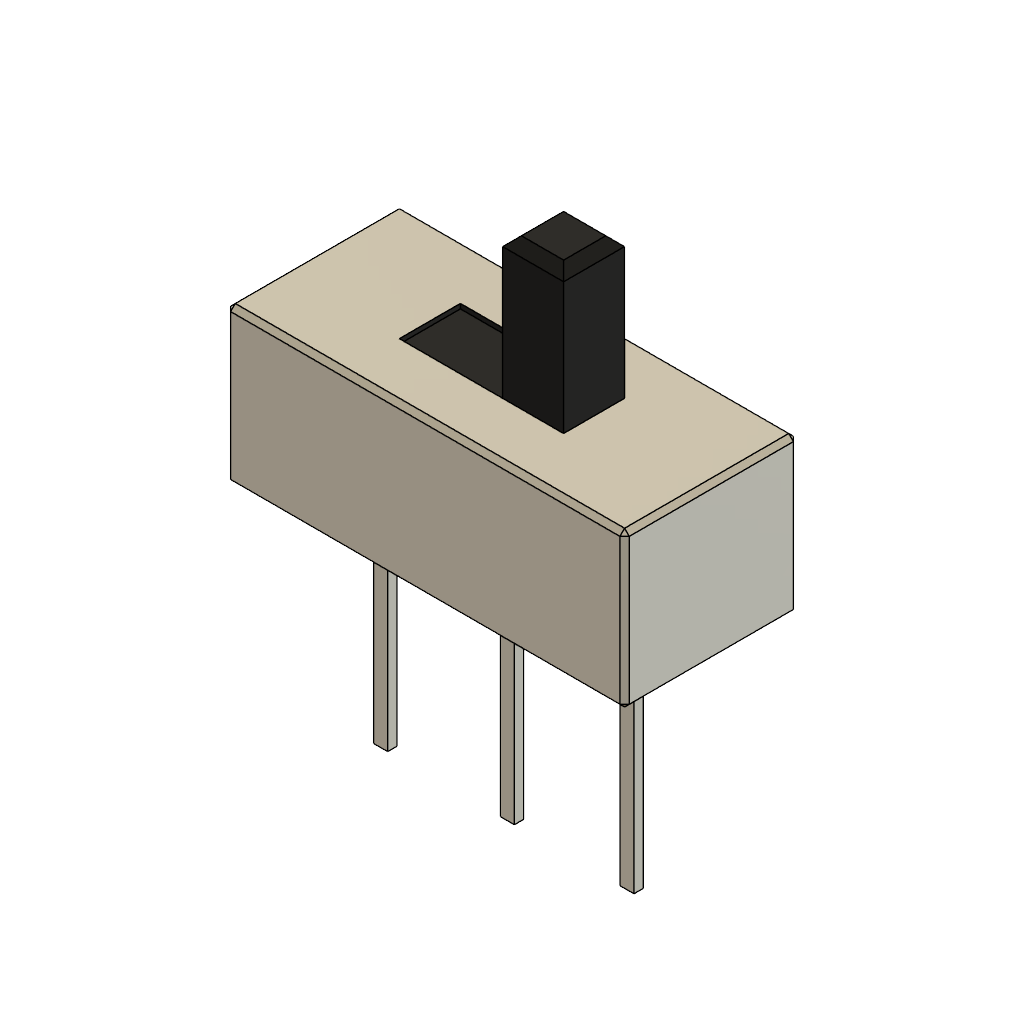
LinearSwitch (Autodesk Fusion 360 design; units mm, degrees)
part number: 2026-08-16-16-37-15-507
Autodesk Fusion 360 part; units mm, degrees
sketch "Sketch1" plane through (0, 0, 0) normal (0, 1, 0) x (1, 0, 0)
  line L0 (4.25, 1.85) -> (-4.25, 1.85)
  line L1 (-4.25, 1.85) -> (-4.25, -1.85)
  line L2 (-4.25, -1.85) -> (4.25, -1.85)
  line L3 (4.25, -1.85) -> (4.25, 1.85)
  line L4 (4.25, 1.85) -> (-4.25, -1.85) construction
  line L5 (-4.25, 1.85) -> (4.25, -1.85) construction
  dimension "d1" = 8.5
  dimension "d2" = 3.7
  constraint horizontal L0
  constraint perpendicular L0 L1
  constraint parallel L0 L2
  constraint parallel L1 L3
  constraint coincident L4 origin
  constraint coincident L5 origin
  measures "d1" distance of L1.end L2.end
  measures "d2" distance of L0.end L1.end
extrude "Extrude1" add sketch "Sketch1" along normal blind 3.3
sketch "Sketch2" plane through (0, 3.3, 0) normal (0, 1, 0) x (-1, 0, 0)
  line L0 (-4.25, 1.85) -> (-4.25, -1.85)
  line L1 (-4.25, -1.85) -> (4.25, -1.85)
  line L2 (4.25, -1.85) -> (4.25, 1.85)
  line L3 (4.25, 1.85) -> (-4.25, 1.85)
  line L4 (-4.25, 0) -> (-1.75, 0)
  line L5 (-1.75, 0) -> (-1.1, 0)
  line L6 (-1.75, -0.65) -> (-0.45, -0.65)
  line L7 (-0.45, -0.65) -> (-0.45, 0.65)
  line L8 (-0.45, 0.65) -> (-1.75, 0.65)
  line L9 (-1.75, 0.65) -> (-1.75, -0.65)
  line L10 (-1.75, -0.65) -> (-0.45, 0.65) construction
  line L11 (-0.45, -0.65) -> (-1.75, 0.65) construction
  line L12 (4.25, 0) -> (1.75, 0)
  line L13 (1.75, 0) -> (1.1, 0)
  line L14 (0.45, -0.65) -> (1.75, -0.65)
  line L15 (1.75, -0.65) -> (1.75, 0.65)
  line L16 (1.75, 0.65) -> (0.45, 0.65)
  line L17 (0.45, 0.65) -> (0.45, -0.65)
  line L18 (0.45, -0.65) -> (1.75, 0.65) construction
  line L19 (1.75, -0.65) -> (0.45, 0.65) construction
  line L20 (0.45, -0.65) -> (-0.45, -0.65)
  line L21 (0.45, 0.65) -> (-0.45, 0.65)
  point P0 (-1.1, 0)
  point P1 (1.1, 0)
  dimension "d5" = 2.5
  dimension "d6" = 0.65
  dimension "d7" = 1.3
  dimension "d8" = 1.3
  dimension "d9" = 2.5
  dimension "d10" = 0.65
  dimension "d11" = 1.3
  dimension "d12" = 1.3
  constraint midpoint L0 L4.start
  constraint perpendicular L0 L4
  constraint parallel L4 L5
  constraint horizontal L6
  constraint perpendicular L6 L7
  constraint parallel L6 L8
  constraint parallel L7 L9
  constraint coincident L10 P0
  constraint coincident L11 P0
  constraint coincident P0 L5.end
  constraint midpoint L2 L12.start
  constraint perpendicular L2 L12
  constraint parallel L12 L13
  constraint horizontal L14
  constraint perpendicular L14 L15
  constraint parallel L14 L16
  constraint parallel L15 L17
  constraint coincident L18 P1
  constraint coincident L19 P1
  constraint coincident P1 L13.end
  measures "d5" distance of L4.start L4.end
  measures "d6" distance of L4.end P0
  measures "d7" distance of L7.end L8.end
  measures "d8" distance of L6.end L7.end
  measures "d9" distance of L12.start L12.end
  measures "d10" distance of L12.end P1
  measures "d11" distance of L15.end L16.end
  measures "d12" distance of L14.end L15.end
extrude "Extrude2" cut sketch "Sketch2" against normal blind 0.1 contours L14 L15 L16 L17 | L7 L17 L20 L21
extrude "Extrude3" add sketch "Sketch2" along normal blind 3 contours L6 L7 L8 L9
chamfer "Chamfer1" distance 0.2 angle 45 4 edges at (1.1, 6.3, 0.65) (0.45, 6.3, 0) (1.1, 6.3, -0.65) (1.75, 6.3, 0)
chamfer "Chamfer2" distance 0.1 angle 45 12 edges at (0, 3.3, 1.85) (4.25, 3.3, 0) (-4.25, 3.3, 0) (0, 3.3, -1.85) (4.25, 1.65, 1.85) (4.25, 1.65, -1.85) (4.25, 0, 0) (0, 0, 1.85) (-4.25, 1.65, 1.85) (-4.25, 1.65, -1.85) (0, 0, -1.85) (-4.25, 0, 0)
sketch "Sketch3" plane through (0, 0, 0) normal (0, -1, 0) x (1, 0, 0)
  line L0 (-4.15, -1.75) -> (4.15, -1.75)
  line L1 (4.15, -1.75) -> (4.15, 1.75)
  line L2 (4.15, 1.75) -> (-4.15, 1.75)
  line L3 (-4.15, 1.75) -> (-4.15, -1.75)
  line L4 (0.15, 0.1) -> (-0.15, 0.1)
  line L5 (-0.15, 0.1) -> (-0.15, -0.1)
  line L6 (-0.15, -0.1) -> (0.15, -0.1)
  line L7 (0.15, -0.1) -> (0.15, 0.1)
  line L8 (0.15, 0.1) -> (-0.15, -0.1) construction
  line L9 (-0.15, 0.1) -> (0.15, -0.1) construction
  line L10 (0, 0) -> (2.7, 0)
  line L11 (2.7, 0) -> (2.55, 0)
  line L12 (2.7, 0.1) -> (2.4, 0.1)
  line L13 (2.4, 0.1) -> (2.4, -0.1)
  line L14 (2.4, -0.1) -> (2.7, -0.1)
  line L15 (2.7, -0.1) -> (2.7, 0.1)
  line L16 (2.7, 0.1) -> (2.4, -0.1) construction
  line L17 (2.4, 0.1) -> (2.7, -0.1) construction
  line L18 (-0.15, 0) -> (-2.85, 0)
  line L19 (-2.85, 0) -> (-2.7, 0)
  line L20 (-2.55, 0.1) -> (-2.85, 0.1)
  line L21 (-2.85, 0.1) -> (-2.85, -0.1)
  line L22 (-2.85, -0.1) -> (-2.55, -0.1)
  line L23 (-2.55, -0.1) -> (-2.55, 0.1)
  line L24 (-2.55, 0.1) -> (-2.85, -0.1) construction
  line L25 (-2.85, 0.1) -> (-2.55, -0.1) construction
  point P0 (2.55, 0)
  point P1 (-2.7, 0)
  dimension "d19" = 0.3
  dimension "d20" = 0.2
  dimension "d23" = 2.7
  dimension "d24" = 0.15
  dimension "d25" = 0.3
  dimension "d26" = 0.2
  dimension "d27" = 2.7
  dimension "d28" = 0.15
  dimension "d29" = 0.3
  dimension "d30" = 0.2
  constraint horizontal L4
  constraint perpendicular L4 L5
  constraint parallel L4 L6
  constraint parallel L5 L7
  constraint coincident L8 L10.start
  constraint coincident L9 L10.start
  constraint coincident L10.start origin
  constraint perpendicular L7 L10
  constraint parallel L10 L11
  constraint horizontal L12
  constraint perpendicular L12 L13
  constraint parallel L12 L14
  constraint parallel L13 L15
  constraint coincident L16 P0
  constraint coincident L17 P0
  constraint coincident P0 L11.end
  constraint midpoint L5 L18.start
  constraint perpendicular L5 L18
  constraint parallel L18 L19
  constraint horizontal L20
  constraint perpendicular L20 L21
  constraint parallel L20 L22
  constraint parallel L21 L23
  constraint coincident L24 P1
  constraint coincident L25 P1
  constraint coincident P1 L19.end
  measures "d19" distance of L5.end L6.end
  measures "d20" distance of L4.end L5.end
  measures "d23" distance of L10.start L10.end
  measures "d24" distance of L10.end P0
  measures "d25" distance of L13.end L14.end
  measures "d26" distance of L12.end L13.end
  measures "d27" distance of L18.start L18.end
  measures "d28" distance of L18.end P1
  measures "d29" distance of L21.end L22.end
  measures "d30" distance of L20.end L21.end
extrude "Extrude4" add sketch "Sketch3" along normal blind 5 contours L4 L5 L6 L7
extrude "Extrude5" add sketch "Sketch3" along normal blind 5 contours L18 L19 L21 L22 L23 | L18 L19 L20 L21 L23
extrude "Extrude6" add sketch "Sketch3" along normal blind 5 contours L10 L11 L12 L13 L15 | L10 L11 L13 L14 L15
